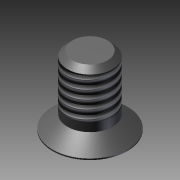
# Autodesk Inventor part: 8-32_1
Saved by Autodesk Inventor 2011 SP1 (Build 150282100, 282)
## iProperties
Created: 2017-08-19
Part Number: 8-32_1
Catalog Web Link: www.cadenas.de
Description: 8-32, 10-24_1-Countersunk Bolt
Vendor: 8020
Document SubType Name: Modeling
Designer: psAdmin
Manufacturer: 8020
Mass: 0.0956613 g
Surface Area: 1.54494 cm^2
Volume: 0.0956613 cm^3
Density: 1 g/cm^3
Category: PARTsolutions
Company: 8020
Title: 8-32_1
Author: Cadenas PARTsolutions
Comments: Countersunk Bolt
PSOL_IDENT_0: {$CADENAS_DATA\23d-libs\8020\inch\linear_motion\csunk_bolt_1.prj},152 {VTYP=3D},{NB=8-32_1},{LINA=8-
PSOL_IDENT_1: 32_1},{NN=8-32, 10-24_1},{DATE=22.08.2012},{GEOMDATE=29.11.2011 06:57:00},{VERSION=},{LINEID=10},{LI
PSOL_IDENT_2: NESUBID=-1},{WBVAR=}  {NB=8-32_1},{LINA=8-32_1},{KT=DUMMY},{PN=8-32},{A=1.000},{TH=0.156},{CS=0.283}
PSOL_IDENT_3: ,{HD1=0.177}
NN: 8-32, 10-24_1
NT: Countersunk Bolt
NB: 8-32_1
NBSYN: $PN._1
LINA: 8-32_1
PN: 8-32
A: 1.000
TH: 0.156
CS: 0.283
HD1: 0.177
SUPPLIER: 8020
ARTICLENO: 8-32_1
BOMINFO: 8-32_1
CREATOR: CADENAS GmbH
Autodesk Inventor part; units mm, degrees
ref_plane "YZ Plane" through (0, 0, 0) normal (1, 0, 0) x (0, 1, 0)
ref_plane "XZ Plane" through (0, 0, 0) normal (0, 1, 0) x (-1, 0, 0)
ref_plane "XY Plane" through (0, 0, 0) normal (0, 0, 1) x (1, 0, 0)
sketch "Sketch_1" plane through (0, 0, 0) normal (0, 0, 1) x (1, 0, 0)
  line L0 (0, -1.1296) -> (0, 5.2204)
  line L1 (0, 5.2204) -> (1.6104, 5.2204)
  line L2 (1.6104, 5.2204) -> (2.0828, 4.748)
  line L3 (2.0828, 4.748) -> (2.0828, 0.1385)
  line L4 (2.0828, 0.1385) -> (3.4503, -1.009)
  line L5 (3.4503, -1.009) -> (3.4503, -1.1296)
  line L6 (3.4503, -1.1296) -> (0, -1.1296)
  line L7 (0, -1.1296) -> (0, 5.2204)
  constraints: 16 end point
revolve "Revolution1" add sketch "Sketch_1" angle 360 about axis through (0, -1.1296, 0) along (0, -1, 0)
thread "Thread1" size "8-32 UNC" class "2A" standard "ANSI Unified Screw Threads" length 3.7911
sketch "Sketch_2" plane through (0, -1.1296, 0) normal (0, -1, 0) x (1, 0, 0)
  line L0 (-1.1906, -0.6874) -> (0, -1.3748)
  line L1 (0, -1.3748) -> (1.1906, -0.6874)
  line L2 (1.1906, -0.6874) -> (1.1906, 0.6874)
  line L3 (1.1906, 0.6874) -> (0, 1.3748)
  line L4 (0, 1.3748) -> (-1.1906, 0.6874)
  line L5 (-1.1906, 0.6874) -> (-1.1906, -0.6874)
  constraints: 12 end point
extrude "Extrusion1" cut sketch "Sketch_2" against normal blind 0.7925
sketch "Sketch_3" plane through (0, 0, 0) normal (0, 0, 1) x (1, 0, 0)
  line L0 (0, -0.3371) -> (0, 0.3503)
  line L1 (0, 0.3503) -> (1.1906, -0.3371)
  line L2 (1.1906, -0.3371) -> (0, -0.3371)
  line L3 (0, -0.3371) -> (0, 0.3503)
  constraints: 8 end point
revolve "Revolution2" cut sketch "Sketch_3" angle 360 about axis through (0, -0.3371, 0) along (0, -1, 0)
ref_plane "screw_XY" through (0, 0, 0) normal (0, 1, 0) x (1, 0, 0)
ref_plane "screw_YZ" through (0, 0, 0) normal (1, 0, 0) x (0, 0, -1)
ref_plane "screw_ZX" through (0, 0, 0) normal (0, 0, -1) x (0, 1, 0)
body "Solid1"
